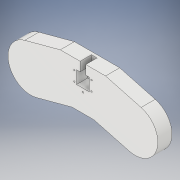
# Autodesk Inventor part: HA002
Saved by Autodesk Inventor 2017 SP1 (Build 210196100, 196)
## iProperties
Created: 2017-06-10
Part Number: HA002
Material: ABS Plastic
Document SubType Name: Modeling
Designer: Zach
Density: 1.06 g/cm^3
Appearance: CR White
Author: Zach
Autodesk Inventor part; units mm, degrees
ref_plane "YZ Plane" through (0, 0, 0) normal (1, 0, 0) x (0, 1, 0)
ref_plane "XZ Plane" through (0, 0, 0) normal (0, 1, 0) x (-1, 0, 0)
ref_plane "XY Plane" through (0, 0, 0) normal (0, 0, 1) x (1, 0, 0)
sketch "Sketch1" plane through (0, 0, 0) normal (0, 0, 1) x (1, 0, 0)
  line L0 (0, 0) -> (160, 0)
  line L1 (160, 0) -> (118.589, -154.5481)
  line L2 (0, 0) -> (41.411, -154.5481)
  line L3 (41.411, -154.5481) -> (118.589, -154.5481)
  dimension "d0" = 160
  dimension "d1" = 160
  dimension "d2" = 160
  dimension "d3" = 75
  dimension "d4" = 75
  constraints: 8 end point, 1 coincident, 1 horizontal
  measures "d0" distance of L0.start L0.end
  measures "d1" distance of L0.end L1.end
  measures "d2" distance of L0.start L2.end
  measures "d3" angle of L0 L1
  measures "d4" angle of L0 L2
extrude "Extrusion1" add sketch "Sketch1" along normal blind 50
sketch "Sketch3" plane through (0, 0, 50) normal (0, 0, 1) x (1, 0, 0)
  line L0 (57.5, -32.2741) -> (102.5, -32.2741)
  line L1 (102.5, -32.2741) -> (102.5, -77.2741)
  line L2 (102.5, -77.2741) -> (57.5, -77.2741)
  line L3 (57.5, -77.2741) -> (57.5, -32.2741)
  line L4 (0, 0) -> (41.411, -154.5481) projected
  line L5 (160, 0) -> (0, 0) projected
  line L6 (70, 0) -> (90, 0)
  line L7 (90, 0) -> (90, -32.2741)
  line L8 (90, -32.2741) -> (70, -32.2741)
  line L9 (70, -32.2741) -> (70, 0)
  point P0 (20.7055, -77.2741)
  point P1 (80, 0)
  point P2 (80, -32.2741)
  point P3 (80, -32.2741)
  point P4 (80, 0)
  dimension "d10" = 45
  dimension "d11" = 45
  dimension "d14" = 20
  constraints: 16 end point, 5 midpoint, 4 parallel, 2 horizontal, 2 horizontal alignment, 2 perpendicular, 2 vertical alignment, 1 point on line
  measures "d10" distance of L1.end L2.end
  measures "d11" distance of L0.end L1.end
  measures "d14" distance of L7.end L8.end
extrude "Extrusion3" cut sketch "Sketch3" against normal blind 40
sketch "Sketch4" plane through (0, 0, 50) normal (0, 0, 1) x (1, 0, 0)
  line L0 (70, -32.2741) -> (70, 0) projected
  line L1 (70, 0) -> (0, 0) projected
  line L2 (0, 0) -> (41.411, -154.5481) projected
  line L3 (41.411, -154.5481) -> (118.589, -154.5481) projected
  line L4 (118.589, -154.5481) -> (160, 0) projected
  line L5 (160, 0) -> (90, 0) projected
  line L6 (90, 0) -> (90, -32.2741) projected
  line L7 (90, -32.2741) -> (102.5, -32.2741) projected
  line L8 (102.5, -32.2741) -> (102.5, -77.2741) construction
  line L9 (102.5, -77.2741) -> (57.5, -77.2741) projected
  line L10 (57.5, -77.2741) -> (57.5, -32.2741) projected
  line L11 (57.5, -32.2741) -> (70, -32.2741) projected
  line L12 (57.5, -77.2741) -> (102.5, -77.2741) construction
  line L13 (102.5, -77.2741) -> (102.5, -32.2741)
  line L14 (102.5, -32.2741) -> (57.5, -32.2741) construction
  line L15 (57.5, -32.2741) -> (57.5, -77.2741) construction
  line L16 (57.5, -77.2741) -> (102.5, -32.2741) construction
  line L17 (102.5, -77.2741) -> (57.5, -32.2741) construction
  circle A0 centre (80, -19.7741) radius 2.5
  circle A1 centre (49.6891, -37.2741) radius 2.5
  circle A2 centre (49.6891, -72.2741) radius 2.5
  circle A3 centre (80, -89.7741) radius 2.5
  circle A4 centre (110.3109, -72.2741) radius 2.5
  circle A5 centre (110.3109, -37.2741) radius 2.5
  point P0 (80, -54.7741)
  point P1 (80, -54.7741)
  dimension "d15" = 45
  dimension "d16" = 45
  dimension "d17" = 5
  dimension "d18" = 35
  dimension "d21" = 360
  constraints: 12 end point, 6 centre point, 3 midpoint, 2 parallel, 1 horizontal, 1 perpendicular, 1 vertical alignment, 13 other
  measures "d15" distance of L10.end L13.end
  measures "d16" distance of L13.end L12.end
  measures "d17" diameter of A0
  measures "d18" distance of point (80, -54.774) A0.centre
extrude "Extrusion4" cut sketch "Sketch4" against normal through all contours A1 | A2 | A3 | A4 | A5
sketch "Sketch5" plane through (0, 0, 50) normal (0, 0, 1) x (1, 0, 0)
  line L0 (160, 0) -> (90, 0) projected
  line L1 (160, 0) -> (285.5704, -33.6465)
  line L2 (118.589, -154.5481) -> (41.411, -154.5481) projected
  line L3 (118.589, -154.5481) -> (244.1593, -188.1946)
  circle A0 centre (264.8648, -110.9205) radius 80 construction
  arc A1 (244.1593, -188.1946) -> (285.5704, -33.6465) centre (264.8648, -110.9205) ccw
  line L4 (160, 0) -> (118.589, -154.5481)
  line L5 (0, 0) -> (41.411, -154.5481) projected
  line L6 (0, 0) -> (-125.5704, -33.6465)
  line L7 (41.411, -154.5481) -> (118.589, -154.5481) projected
  line L8 (41.411, -154.5481) -> (-84.1593, -188.1946)
  circle A2 centre (-104.8648, -110.9205) radius 80 construction
  arc A3 (-125.5704, -33.6465) -> (-84.1593, -188.1946) centre (-104.8648, -110.9205) ccw
  dimension "d25" = 130
  dimension "d26" = 130
  dimension "d27" = 160
  dimension "d30" = 130
  dimension "d31" = 130
  dimension "d32" = 160
  constraints: 10 end point, 8 point on circle, 6 tangent, 4 centre point, 1 concentric
  measures "d25" distance of L0.start L1.end
  measures "d26" distance of L2.start L3.end
  measures "d27" diameter of A0
  measures "d30" distance of L5.start L6.end
  measures "d31" distance of L2.end L8.end
  measures "d32" diameter of A2
extrude "Extrusion5" add sketch "Sketch5" against normal blind 50
body "Solid1"
